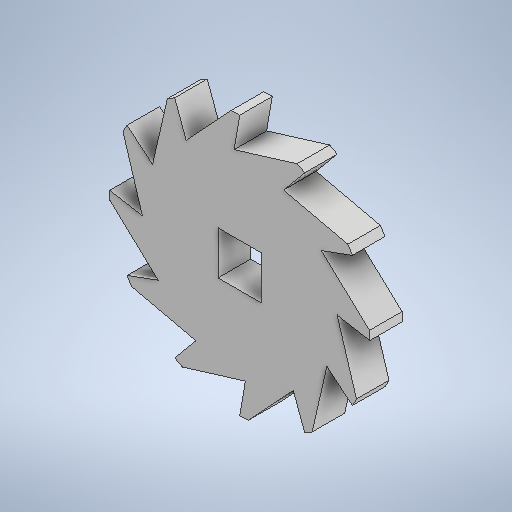
# Autodesk Inventor part: Pieza 3
Saved by Autodesk Inventor 2025.3 (Build 293356030, 356C)
## iProperties
Created: 2025-08-24
Part Number: Pieza 3
Material: Generic
Document SubType Name: Modeling
Designer: PC
Density: 1 g/cm^3
Appearance: Default
Author: PC
Autodesk Inventor part; units mm, degrees
ref_plane "YZ Plane" through (0, 0, 0) normal (1, 0, 0) x (0, 1, 0)
ref_plane "XZ Plane" through (0, 0, 0) normal (0, 1, 0) x (-1, 0, 0)
ref_plane "XY Plane" through (0, 0, 0) normal (0, 0, 1) x (1, 0, 0)
sketch "Sketch1" plane through (0, 0, 0) normal (0, 0, 1) x (1, 0, 0)
  circle A0 centre (0, 0) radius 22.5 construction
  line L0 (0, 0) -> (0, 37.8741) construction
  line L1 (0, 0) -> (16.9755, 34.5141) construction
  line L2 (0, 0) -> (38.4628, 0) construction
  line L3 (13.2405, 26.9201) -> (-1.3032, 22.4622)
  line L4 (0, 30) -> (-1.3032, 22.4622)
  line L5 (-1.9934, 29.9337) -> (-12.3597, 18.8012)
  line L6 (-15, 25.9808) -> (-12.3597, 18.8012)
  line L7 (-16.6932, 24.9266) -> (-20.1045, 10.1025)
  line L8 (-25.9808, 15) -> (-20.1045, 10.1025)
  line L9 (-26.9201, 13.2405) -> (-22.4622, -1.3032)
  line L10 (-30, 0) -> (-22.4622, -1.3032)
  line L11 (-29.9337, -1.9934) -> (-18.8012, -12.3597)
  line L12 (-25.9808, -15) -> (-18.8012, -12.3597)
  line L13 (-24.9266, -16.6932) -> (-10.1025, -20.1045)
  line L14 (-15, -25.9808) -> (-10.1025, -20.1045)
  line L15 (-13.2405, -26.9201) -> (1.3032, -22.4622)
  line L16 (0, -30) -> (1.3032, -22.4622)
  line L17 (1.9934, -29.9337) -> (12.3597, -18.8012)
  line L18 (15, -25.9808) -> (12.3597, -18.8012)
  line L19 (16.6932, -24.9266) -> (20.1045, -10.1025)
  line L20 (25.9808, -15) -> (20.1045, -10.1025)
  line L21 (26.9201, -13.2405) -> (22.4622, 1.3032)
  line L22 (30, 0) -> (22.4622, 1.3032)
  line L23 (29.9337, 1.9934) -> (18.8012, 12.3597)
  line L24 (25.9808, 15) -> (18.8012, 12.3597)
  line L25 (24.9266, 16.6932) -> (10.1025, 20.1045)
  line L26 (15, 25.9808) -> (10.1025, 20.1045)
  arc A1 (-15, 25.9808) -> (-16.6932, 24.9266) centre (0, 0) ccw
  arc A2 (-25.9808, 15) -> (-26.9201, 13.2405) centre (0, 0) ccw
  arc A3 (-30, 0) -> (-29.9337, -1.9934) centre (0, 0) ccw
  arc A4 (-25.9808, -15) -> (-24.9266, -16.6932) centre (0, 0) ccw
  arc A5 (-15, -25.9808) -> (-13.2405, -26.9201) centre (0, 0) ccw
  arc A6 (0, -30) -> (1.9934, -29.9337) centre (0, 0) ccw
  arc A7 (15, -25.9808) -> (16.6932, -24.9266) centre (0, 0) ccw
  arc A8 (25.9808, -15) -> (26.9201, -13.2405) centre (0, 0) ccw
  arc A9 (30, 0) -> (29.9337, 1.9934) centre (0, 0) ccw
  arc A10 (25.9808, 15) -> (24.9266, 16.6932) centre (0, 0) ccw
  arc A11 (15, 25.9808) -> (13.2405, 26.9201) centre (0, 0) ccw
  arc A12 (0, 30) -> (-1.9934, 29.9337) centre (0, 0) ccw
  line L27 (5, -5) -> (-5, -5)
  line L28 (-5, -5) -> (-5, 5)
  line L29 (-5, 5) -> (5, 5)
  line L30 (5, 5) -> (5, -5)
  line L31 (5, -5) -> (-5, 5) construction
  line L32 (-5, -5) -> (5, 5) construction
  dimension "d0" = 45
  dimension "d2" = 63.81
  dimension "d3" = 63.15
  dimension "d6" = 360
  dimension "d8" = 10
  dimension "d9" = 10
  constraints: 66 end point, 24 point on circle, 12 centre point, 2 coincident, 2 horizontal, 2 midpoint, 2 parallel, 2 point on line, 1 equal length, 1 perpendicular, 1 vertical, 64 other
  measures "d2" angle of L2 L1
  measures "d3" angle of L3 L4
  measures "d8" distance of L28.end L29.end
  measures "d9" distance of L27.end L28.end
extrude "Extrusion1" add sketch "Sketch1" along normal blind 7.5
body "Solid1"
